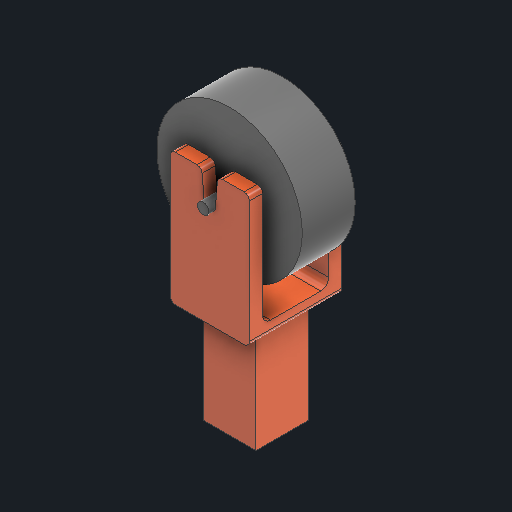
# Autodesk Inventor part: RouleauTendeur
Saved by Autodesk Inventor 2026.2 (Build 302298010, 298A)
## iProperties
Created: 2026-04-13
Part Number: RouleauTendeur
Material: Générique
Document SubType Name: Modeling
Designer: romai
Density: 1 g/cm^3
Appearance: Par défaut
Author: romai
Autodesk Inventor part; units mm, degrees
ref_plane "YZ Plane" through (0, 0, 0) normal (1, 0, 0) x (0, 1, 0)
ref_plane "XZ Plane" through (0, 0, 0) normal (0, 1, 0) x (-1, 0, 0)
ref_plane "XY Plane" through (0, 0, 0) normal (0, 0, 1) x (1, 0, 0)
sketch "Esquisse2" plane through (0, 0, 0) normal (0, 1, 0) x (-1, 0, 0)
  line L0 (10, -10) -> (-10, -10)
  line L1 (-10, -10) -> (-10, 10)
  line L2 (-10, 10) -> (10, 10)
  line L3 (10, 10) -> (10, -10)
  line L4 (10, -10) -> (-10, 10) construction
  line L5 (-10, -10) -> (10, 10) construction
  point P0 (0, 0)
  dimension "d6" = 20
  dimension "d7" = 20
  constraints: 12 end point, 2 midpoint, 2 parallel, 1 horizontal, 1 perpendicular
  measures "d6" distance of L1.end L2.end
  measures "d7" distance of L0.end L1.end
extrude "Extrusion1" add sketch "Esquisse2" along normal blind 40
sketch "Esquisse3" plane through (0, 0, 0) normal (0, 0, 1) x (1, 0, 0)
  line L0 (-10, 40) -> (10, 40) projected
  line L1 (15, 88) -> (15, 42)
  line L2 (13, 40) -> (-13, 40)
  line L3 (-15, 42) -> (-15, 88)
  line L4 (-15, 90) -> (15, 40) construction
  line L5 (15, 90) -> (-15, 40) construction
  line L6 (13, 90) -> (4.8464, 90)
  line L7 (-4.8464, 90) -> (-13, 90)
  line L8 (-15, 90) -> (-3, 90)
  line L9 (3, 90) -> (15, 90)
  line L10 (-2.8528, 88.1595) -> (-2.1472, 79.3405)
  line L11 (-0.1536, 77.5) -> (0.1536, 77.5)
  line L12 (2.1472, 79.3405) -> (2.8528, 88.1595)
  arc A0 (-13, 90) -> (-15, 88) centre (-13, 88) ccw
  arc A1 (15, 88) -> (13, 90) centre (13, 88) ccw
  arc A2 (-2.1472, 79.3405) -> (-0.1536, 77.5) centre (-0.1536, 79.5) ccw
  arc A3 (0.1536, 77.5) -> (2.1472, 79.3405) centre (0.1536, 79.5) ccw
  arc A4 (-2.8528, 88.1595) -> (-4.8464, 90) centre (-4.8464, 88) ccw
  arc A5 (4.8464, 90) -> (2.8528, 88.1595) centre (4.8464, 88) ccw
  arc A6 (-15, 42) -> (-13, 40) centre (-13, 42) ccw
  arc A7 (13, 40) -> (15, 42) centre (13, 42) ccw
  point P0 (0, 0)
  point P1 (0, 65)
  point P2 (-2, 77.5)
  point P3 (2, 77.5)
  dimension "d10" = 30
  dimension "d11" = 50
  dimension "d12" = 0
  dimension "d23" = 12
  dimension "d24" = 12
  dimension "d27" = 4
  dimension "d28" = 1
  dimension "d29" = 37.5
  dimension "d30" = 2
  constraints: 24 end point, 16 point on circle, 16 point on line, 16 tangent, 8 centre point, 7 equal radius, 3 horizontal, 3 parallel, 3 perpendicular, 2 collinear, 2 midpoint
  measures "d10" distance of L4.end L5.end
  measures "d11" distance of L5.start L4.end
  measures "d12" distance between parallel lines of L0 L2
  measures "d23" distance of L5.start L9.start
  measures "d24" distance of L8.end L4.start
  measures "d27" distance of point (-2, 77.5) point (2, 77.5)
  measures "d28" horizontal distance of L8.end point (-2, 77.5)
  measures "d29" distance between parallel lines of L0 L11
  measures "d30" radius of A0
extrude "Extrusion2" add sketch "Esquisse3" along normal mid plane 35
sketch "Esquisse5" plane through (15, 42, 17.5) normal (1, 0, 0) x (0, 0, -1)
  line L0 (5, 61.6074) -> (30, 61.6074)
  line L1 (30, 61.6074) -> (30, 6)
  line L2 (27, 3) -> (8, 3)
  line L3 (5, 6) -> (5, 61.6074)
  line L4 (5, 61.6074) -> (30, 3) construction
  line L5 (30, 61.6074) -> (5, 3) construction
  line L6 (35, 46) -> (35, 0) projected
  line L7 (35, -2) -> (0, -2) projected
  line L8 (0, 0) -> (0, 46) projected
  arc A0 (5, 6) -> (8, 3) centre (8, 6) ccw
  arc A1 (27, 3) -> (30, 6) centre (27, 6) ccw
  point P0 (17.5, -42)
  point P1 (17.5, 32.3037)
  dimension "d31" = 5
  dimension "d32" = 5
  dimension "d33" = 5
  dimension "d34" = 3
  constraints: 12 end point, 4 point on circle, 4 point on line, 4 tangent, 2 centre point, 2 midpoint, 2 parallel, 1 equal radius, 1 horizontal, 1 perpendicular
  measures "d31" distance between parallel lines of L6 L1
  measures "d32" distance between parallel lines of L7 L2
  measures "d33" distance between parallel lines of L8 L3
  measures "d34" radius of A0
extrude "Extrusion4" cut sketch "Esquisse5" against normal blind 35
sketch "Esquisse6" plane through (0, 0, 0) normal (0, 0, 1) x (1, 0, 0)
  circle A0 centre (0, 80) radius 27.5
  line L0 (13, 40) -> (-13, 40) projected
  point P0 (0, 0)
  dimension "d37" = 55
  dimension "d38" = 40
  constraints: 1 centre point
  measures "d37" diameter of A0
  measures "d38" distance from line of L0 A0.centre
extrude "Extrusion5" add sketch "Esquisse6" along normal mid plane 20
sketch "Esquisse7" plane through (0, 80, -10) normal (0, 0, -1) x (-1, 0, 0)
  circle A0 centre (0, -0.6595) radius 2.1404
  line L0 (-2.1472, -0.6595) -> (-2.8528, 8.1595) projected
  point P0 (0, -80)
  constraints: 1 centre point, 1 tangent
extrude "Extrusion6" add sketch "Esquisse7" along normal blind 10 and the other way blind 30
